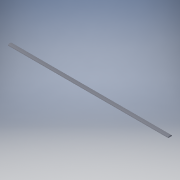
# Autodesk Inventor part: LED light strip
Saved by Autodesk Inventor 2016 (Build 200138000, 138)
## iProperties
Created: 2017-11-04
Part Number: LED light strip
Material: Wood (Cherry)
Document SubType Name: Modeling
Designer: mathaetaes
Density: 0.63 g/cm^3
Appearance: LED Light
Author: mathaetaes
Autodesk Inventor part; units mm, degrees
ref_plane "YZ Plane" through (0, 0, 0) normal (1, 0, 0) x (0, 1, 0)
ref_plane "XZ Plane" through (0, 0, 0) normal (0, 1, 0) x (-1, 0, 0)
ref_plane "XY Plane" through (0, 0, 0) normal (0, 0, 1) x (1, 0, 0)
sketch "Sketch1" plane through (0, 0, 0) normal (0, 1, 0) x (-1, 0, 0)
  line L0 (360.8724, 2.8366) -> (-45.5276, 2.8366)
  line L1 (-45.5276, 2.8366) -> (-45.5276, -6.6884)
  line L2 (-45.5276, -6.6884) -> (360.8724, -6.6884)
  line L3 (360.8724, -6.6884) -> (360.8724, 2.8366)
  point P0 (0, 0)
  dimension "d0" = 406.4
  dimension "d1" = 9.525
  constraints: 8 end point, 2 parallel, 1 horizontal, 1 perpendicular
  measures "d0" distance of L2.end L1.end
  measures "d1" distance of L1.end L0.end
extrude "Extrusion1" add sketch "Sketch1" along normal blind 3.175
fillet "Fillet1" radius 3.175 2 edges at (-157.6724, 3.175, 2.8366) (-157.6724, 3.175, -6.6884)
body "Solid1"
